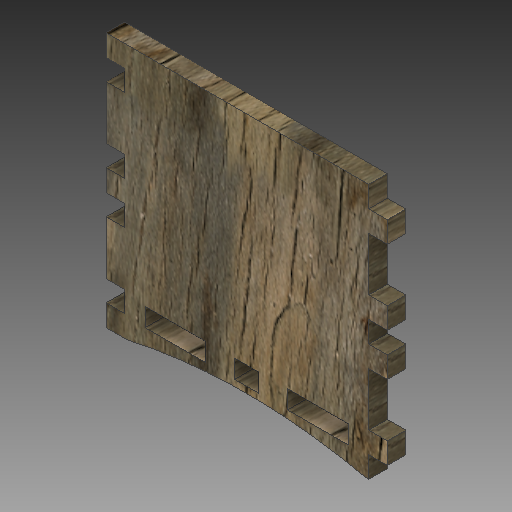
# Autodesk Inventor part: CandleHolder-2
Saved by Autodesk Inventor 2017 (Build 210142000, 142)
## iProperties
Created: 2016-10-20
Part Number: CandleHolder-2
Material: Wood (Birch)
Document SubType Name: Modeling
Designer: andrew
Density: 0.55 g/cm^3
Appearance: Driftwood
Author: andrew
Autodesk Inventor part; units mm, degrees
ref_plane "YZ Plane" through (0, 0, 0) normal (1, 0, 0) x (0, 1, 0)
ref_plane "XZ Plane" through (0, 0, 0) normal (0, 1, 0) x (-1, 0, 0)
ref_plane "XY Plane" through (0, 0, 0) normal (0, 0, 1) x (1, 0, 0)
sketch "Sketch1" plane through (0, 0, 0) normal (0, 0, 1) x (1, 0, 0)
  line L0 (-46.101, -41.8465) -> (-39.116, -41.8465)
  line L1 (46.101, -41.8465) -> (46.101, -34.8721)
  line L2 (46.101, 41.8465) -> (-46.101, 41.8465)
  line L3 (-46.101, 41.8465) -> (-46.101, 34.8721)
  line L4 (-46.101, -41.8465) -> (46.101, 41.8465) construction
  line L5 (46.101, -41.8465) -> (-46.101, 41.8465) construction
  line L6 (-40.005, 41.8465) -> (-40.005, 34.8721) construction
  line L7 (40.005, -41.8465) -> (40.005, -34.8721)
  line L8 (-40.005, -29.4005) -> (-33.3375, -29.4005) construction
  line L9 (-40.005, -35.4965) -> (-33.3375, -35.4965) construction
  line L10 (-33.3375, -29.4005) -> (-33.3375, -35.4965) construction
  line L11 (-13.335, -29.4005) -> (-13.335, -35.4965) construction
  line L12 (-33.3375, -29.4005) -> (-13.335, -29.4005) construction
  line L13 (-13.335, -29.4005) -> (-4.0005, -29.4005) construction
  line L14 (-13.335, -35.4965) -> (-4.0005, -35.4965) construction
  line L15 (-33.3375, -35.4965) -> (-13.335, -35.4965) construction
  line L16 (-64.5414, 0) -> (64.5414, 0) construction
  line L17 (-46.101, 34.8721) -> (-40.005, 34.8721) construction
  line L18 (-46.101, 27.8977) -> (-40.005, 27.8977) construction
  line L19 (40.005, 34.8721) -> (46.101, 34.8721)
  line L20 (-46.101, 34.8721) -> (-46.101, 34.8086)
  line L21 (-46.101, 27.8977) -> (-46.101, 10.3981)
  line L22 (-40.005, 34.8721) -> (-40.005, 27.8977) construction
  line L23 (-40.005, 27.8977) -> (-40.005, 10.4616) construction
  line L24 (46.101, 34.8721) -> (46.101, 41.8465)
  line L25 (40.005, 34.8721) -> (40.005, 41.8465)
  line L26 (-33.274, -35.4648) -> (-13.3985, -35.4648)
  line L27 (-13.3985, -35.4648) -> (-13.3985, -29.4323)
  line L28 (-13.3985, -29.4323) -> (-33.274, -29.4323)
  line L29 (-33.274, -29.4323) -> (-33.274, -35.4648)
  line L30 (-33.274, -35.4648) -> (-13.3985, -29.4323) construction
  line L31 (-13.3985, -35.4648) -> (-33.274, -29.4323) construction
  line L32 (-23.3362, -32.4485) -> (-23.3362, -29.4005) construction
  line L33 (-23.3362, -32.4485) -> (-13.335, -32.4485) construction
  line L34 (-46.101, 34.8086) -> (-40.0367, 34.8086)
  line L35 (-40.0367, 34.8086) -> (-40.0367, 27.9612)
  line L36 (-40.0367, 27.9612) -> (-46.101, 27.9612)
  line L37 (-40.0367, 31.3849) -> (-40.005, 31.3849) construction
  line L38 (-46.101, 34.8086) -> (-46.101, 27.9612)
  line L39 (-46.101, 27.9612) -> (-46.101, 27.8977)
  arc A0 (39.116, -41.8465) -> (-39.116, -41.8465) centre (0, -215.2904) ccw
  line L40 (0, 93.2739) -> (0, -266.7178) construction
  line L41 (-39.116, -41.8465) -> (39.116, -41.8465)
  line L42 (39.116, -41.8465) -> (40.005, -41.8465)
  line L43 (-4.0005, -29.4005) -> (-4.0005, -35.4965) construction
  line L44 (4.0005, -29.4005) -> (4.0005, -35.4965) construction
  line L45 (13.335, -29.4005) -> (13.335, -35.4965) construction
  line L46 (33.3375, -29.4005) -> (33.3375, -35.4965) construction
  line L47 (-3.937, -35.4648) -> (3.937, -35.4648)
  line L48 (3.937, -35.4648) -> (3.937, -29.4323)
  line L49 (3.937, -29.4323) -> (-3.937, -29.4323)
  line L50 (-3.937, -29.4323) -> (-3.937, -35.4648)
  line L51 (-3.937, -35.4648) -> (3.937, -29.4323) construction
  line L52 (3.937, -35.4648) -> (-3.937, -29.4323) construction
  line L53 (13.3985, -35.4648) -> (33.274, -35.4648)
  line L54 (33.274, -35.4648) -> (33.274, -29.4323)
  line L55 (33.274, -29.4323) -> (13.3985, -29.4323)
  line L56 (13.3985, -29.4323) -> (13.3985, -35.4648)
  line L57 (13.3985, -35.4648) -> (33.274, -29.4323) construction
  line L58 (33.274, -35.4648) -> (13.3985, -29.4323) construction
  line L59 (-4.0005, -35.4965) -> (4.0005, -35.4965) construction
  line L60 (4.0005, -35.4965) -> (13.335, -35.4965) construction
  line L61 (4.0005, -29.4005) -> (13.335, -29.4005) construction
  line L62 (-4.0005, -29.4005) -> (4.0005, -29.4005) construction
  line L63 (13.335, -29.4005) -> (33.3375, -29.4005) construction
  line L64 (33.3375, -29.4005) -> (40.005, -29.4005) construction
  line L65 (33.3375, -35.4965) -> (40.005, -35.4965) construction
  line L66 (13.335, -35.4965) -> (33.3375, -35.4965) construction
  line L67 (23.3362, -29.4005) -> (23.3362, -32.4485) construction
  line L68 (-46.101, 10.4616) -> (-40.005, 10.4616) construction
  line L69 (-46.101, 3.4872) -> (-40.005, 3.4872) construction
  line L70 (-46.101, -3.4872) -> (-40.005, -3.4872) construction
  line L71 (-46.101, -10.4616) -> (-40.005, -10.4616) construction
  line L72 (-46.101, -27.8977) -> (-40.005, -27.8977) construction
  line L73 (-46.101, -34.8721) -> (-40.005, -34.8721) construction
  line L74 (-46.101, 10.3981) -> (-40.0367, 10.3981)
  line L75 (-40.0367, 10.3981) -> (-40.0367, 3.5507)
  line L76 (-40.0367, 3.5507) -> (-46.101, 3.5507)
  line L77 (-46.101, -3.5507) -> (-40.0367, -3.5507)
  line L78 (-40.0367, -3.5507) -> (-40.0367, -10.3981)
  line L79 (-40.0367, -10.3981) -> (-46.101, -10.3981)
  line L80 (-46.101, -27.9612) -> (-40.0367, -27.9612)
  line L81 (-40.0367, -27.9612) -> (-40.0367, -34.8086)
  line L82 (-40.0367, -34.8086) -> (-46.101, -34.8086)
  line L83 (-40.005, 10.4616) -> (-40.005, 3.4872) construction
  line L84 (-40.005, 3.4872) -> (-40.005, -3.4872) construction
  line L85 (-40.005, -3.4872) -> (-40.005, -10.4616) construction
  line L86 (-40.005, -10.4616) -> (-40.005, -27.8977) construction
  line L87 (-40.005, -34.8721) -> (-40.005, -41.8465) construction
  line L88 (-40.005, -27.8977) -> (-40.005, -34.8721) construction
  line L89 (-40.0367, -31.3849) -> (-40.005, -31.3849) construction
  line L90 (-40.0367, -6.9744) -> (-40.005, -6.9744) construction
  line L91 (-40.0367, 6.9744) -> (-40.005, 6.9744) construction
  line L92 (-46.101, 10.3981) -> (-46.101, 3.5507)
  line L93 (-46.101, 3.5507) -> (-46.101, -3.5507)
  line L94 (-46.101, -10.3981) -> (-46.101, -27.9612)
  line L95 (-46.101, -3.5507) -> (-46.101, -10.3981)
  line L96 (-46.101, -34.8086) -> (-46.101, -41.8465)
  line L97 (-46.101, -27.9612) -> (-46.101, -34.8086)
  line L98 (46.101, 27.8977) -> (40.005, 27.8977)
  line L99 (40.005, 3.4872) -> (46.101, 3.4872)
  line L100 (40.005, -3.4872) -> (46.101, -3.4872)
  line L101 (40.005, -10.4616) -> (46.101, -10.4616)
  line L102 (40.005, -27.8977) -> (46.101, -27.8977)
  line L103 (40.005, 10.4616) -> (46.101, 10.4616)
  line L104 (40.005, -34.8721) -> (46.101, -34.8721)
  line L105 (40.005, -27.8977) -> (40.005, -10.4616)
  line L106 (40.005, -34.8721) -> (40.005, -27.8977) construction
  line L107 (40.005, -10.4616) -> (40.005, -3.4872) construction
  line L108 (40.005, -3.4872) -> (40.005, 3.4872)
  line L109 (40.005, 3.4872) -> (40.005, 10.4616) construction
  line L110 (40.005, 10.4616) -> (40.005, 27.8977)
  line L111 (40.005, 27.8977) -> (40.005, 34.8721) construction
  line L112 (40.005, -41.8465) -> (46.101, -41.8465)
  line L113 (46.101, -34.8721) -> (46.101, -27.8977)
  line L114 (46.101, -27.8977) -> (46.101, -10.4616)
  line L115 (46.101, -10.4616) -> (46.101, -3.4872)
  line L116 (46.101, -3.4872) -> (46.101, 3.4872)
  line L117 (46.101, 3.4872) -> (46.101, 10.4616)
  line L118 (46.101, 10.4616) -> (46.101, 27.8977)
  line L119 (46.101, 27.8977) -> (46.101, 34.8721)
  point P0 (0, 0)
  point P1 (0, -32.4485)
  dimension "d1" = 6.096
  dimension "d3" = 6.096
  dimension "d4" = 6.35
  dimension "d5" = 20.0025
  dimension "d6" = 13.335
  dimension "d9" = 83.693
  dimension "d10" = 6.9744
  dimension "d11" = 71.247
  dimension "d12" = 6.9744
  dimension "d32" = 6.0325
  dimension "d33" = 19.8755
  dimension "d34" = 6.8474
  dimension "d36" = 6.0643
  dimension "d38" = 6.985
  dimension "d39" = 177.8
  dimension "d40" = 8.001
  dimension "d41" = 4.0005
  dimension "d42" = 20.0025
  dimension "d43" = 7.874
  dimension "d44" = 19.8755
  dimension "d45" = 13.335
  dimension "d46" = 6.9744
  dimension "d47" = 6.9744
  dimension "d48" = 6.8474
  dimension "d49" = 6.8474
  dimension "d50" = 6.8474
  dimension "d51" = 80.01
  dimension "d52" = 6.096
  constraints: 316 perpendicular, 224 end point, 90 parallel, 75 point on line, 58 horizontal, 27 vertical, 20 midpoint, 12 collinear, 2 point on circle, 1 centre point, 70 other
  measures "d1" distance between parallel lines of L9 L8
  measures "d3" distance between parallel lines of L6 L3
  measures "d4" distance between parallel lines of L0 L9
  measures "d5" distance of L8.end L11.start
  measures "d6" distance from line of L11 point (0, 0)
  measures "d9" distance between parallel lines of L2 L0
  measures "d10" distance between parallel lines of L2 L19
  measures "d11" distance between parallel lines of L13 L2
  measures "d12" distance of L3.end L18.start
  measures "d32" distance of L26.end L27.end
  measures "d33" distance of L27.end L28.end
  measures "d34" distance of L34.end L35.end
  measures "d36" distance of L20.end L34.end
  measures "d39" radius of A0
  measures "d40" distance between parallel lines of L44 L43
  measures "d41" distance between parallel lines of L44 L40
  measures "d42" distance between parallel lines of L46 L45
  measures "d43" distance of L48.end L49.end
  measures "d44" distance of L54.end L55.end
  measures "d45" distance between parallel lines of L45 L40
  measures "d46" distance between parallel lines of L69 L68
  measures "d47" distance between parallel lines of L70 L69
  measures "d48" distance between parallel lines of L76 L74
  measures "d49" distance of L77.end L78.end
  measures "d50" distance of L80.end L81.end
  measures "d51" distance of L25.end L6.start
extrude "Extrusion1" add sketch "Sketch1" along normal blind 6.096 contours L96 L82 L81 L80 L94 L79 L78 L77 L93 L76 L75 L74 L21 L39 L36 L35 L34 L20 L3 L2 L25 L19 L119 L98 L110 L103 L117 L99 L108 L100 L115 L101 L105 L102 L113 L104 L7 L42 A0 L0 | L38 L34 L35 L36 | L19 L25 L2 L24 | L29 L28 L27 L26 | L50 L49 L48 L47 | L56 L55 L54 L53
extrude "Extrusion2" cut sketch "Sketch1" along normal blind 6.096 contours L19 L25 L2 L24
extrude "Extrusion3" cut sketch "Sketch1" along normal blind 6.096 contours L38 L34 L35 L36
extrude "Extrusion4" cut sketch "Sketch1" along normal blind 6.096 contours L29 L28 L27 L26 | L50 L49 L48 L47 | L56 L55 L54 L53
fillet "Fillet1" [suppressed]
fillet "Fillet2" [suppressed]
equation "\"d1\" = woodThickness"
equation "\"d3\" = woodThickness"
equation "\"d5\" = toothLength"
equation "\"d6\" = toothOffset"
equation "\"d10\" = 0.0833333 * d9"
equation "\"d11\" = glassHeight - lip"
equation "\"d12\" = d10"
equation "\"d32\" = d1 - lasorTol"
equation "\"d33\" = d5 - 2 * lasorTol"
equation "\"d34\" = d12 - 2 * lasorTol"
equation "\"d36\" = d3 - 0.5 * lasorTol"
equation "\"d40\" = 0.4 * toothLength"
equation "\"d41\" = 0.5 * d40"
equation "\"d42\" = d5"
equation "\"d43\" = d40 - 2 * lasorTol"
equation "\"d44\" = d42 - 2 * lasorTol"
equation "\"d45\" = d6"
equation "\"d46\" = d12"
equation "\"d47\" = d10"
equation "\"d48\" = d34"
equation "\"d49\" = d34"
equation "\"d50\" = d34"
equation "\"d51\" = baseLength"
equation "\"d52\" = woodThickness"
equation "\"d13\" = woodThickness"
equation "\"d15\" = woodThickness"
equation "\"d17\" = woodThickness"
equation "\"d19\" = woodThickness"
equation "\"woodThickness\" = 6.096"
equation "\"toothLength\" = 20.0025"
equation "\"glassHeight\" = 80.772"
equation "\"lip\" = 9.525"
equation "\"lasorTol\" = 0.0635"
equation "\"baseLength\" = 80.01"
equation "\"toothOffset\" = 13.335"
body "Solid1"
